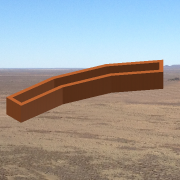
# Autodesk Inventor part: planter
Saved by Autodesk Inventor 2013 SP2 (Build 170200200, 200)
## iProperties
Created: 2014-01-03
Part Number: planter
Material: Wood (Cherry)
Document SubType Name: Modeling
Designer: Dave
Mass: 299055 g
Surface Area: 63083.1 cm^2
Volume: 598109 cm^3
Density: 0.5 g/cm^3
Author: Dave
Autodesk Inventor part; units mm, degrees
ref_plane "YZ Plane" through (0, 0, 0) normal (1, 0, 0) x (0, 1, 0)
ref_plane "XZ Plane" through (0, 0, 0) normal (0, 1, 0) x (-1, 0, 0)
ref_plane "XY Plane" through (0, 0, 0) normal (0, 0, 1) x (1, 0, 0)
sketch "Sketch3" plane through (0, 0, 0) normal (0, 1, 0) x (-1, 0, 0)
  line L0 (4876.8, 0) -> (4710.6271, -1262.2087)
  line L1 (4710.6271, -1262.2087) -> (4223.4327, -2438.4)
  line L2 (4223.4327, -2438.4) -> (3448.4184, -3448.4184)
  line L3 (3122.3395, -3122.3395) -> (3824.0693, -2207.8274)
  line L4 (3824.0693, -2207.8274) -> (4265.195, -1142.8556)
  line L5 (4265.195, -1142.8556) -> (4415.6548, 0)
  line L6 (4876.8, 0) -> (4415.6548, 0)
  line L7 (3448.4184, -3448.4184) -> (3122.3395, -3122.3395)
  line L8 (4776.121, 90.6289) -> (4876.8, 0)
  line L9 (3448.4184, -3448.4184) -> (3245.8, -3603.8929)
  point P0 (0, 0)
  point P1 (0, 0)
  dimension "d20" = 4876.8
  dimension "d25" = 457.2
  constraints: 20 end point, 2 point on line, 1 coincident, 1 horizontal, 8 other
  measures "d20" distance of L0.start point (0, 0)
  measures "d25" distance between parallel lines of L5 L0
extrude "Extrusion1" add sketch "Sketch3" along normal blind 457.2
sketch "Sketch4" plane through (0, 457.2, 0) normal (0, 1, 0) x (1, 0, 0)
  line L0 (-4710.6271, 1262.2087) -> (-4876.8, 0) projected
  line L1 (-4876.8, 0) -> (-4415.6548, 0) projected
  line L2 (-4415.6548, 0) -> (-4265.195, 1142.8556) projected
  line L3 (-4265.195, 1142.8556) -> (-3824.0693, 2207.8274) projected
  line L4 (-3824.0693, 2207.8274) -> (-3122.3395, 3122.3395) projected
  line L5 (-3122.3395, 3122.3395) -> (-3448.4184, 3448.4184) projected
  line L6 (-3448.4184, 3448.4184) -> (-4223.4327, 2438.4) projected
  line L7 (-4223.4327, 2438.4) -> (-4710.6271, 1262.2087) projected
  line L8 (-4145.7787, 2393.5664) -> (-3439.6, 3313.8764)
  line L9 (-3439.6, 3313.8764) -> (-3240.3296, 3114.606)
  line L10 (-3240.3296, 3114.606) -> (-3901.7233, 2252.661)
  line L11 (-3901.7233, 2252.661) -> (-4351.8068, 1166.0631)
  line L12 (-4351.8068, 1166.0631) -> (-4493.618, 88.9)
  line L13 (-4493.618, 88.9) -> (-4775.429, 88.9)
  line L14 (-4775.429, 88.9) -> (-4624.0153, 1239.0012)
  line L15 (-4624.0153, 1239.0012) -> (-4145.7787, 2393.5664)
  point P0 (0, 0)
  dimension "d24" = 88.9
  constraints: 16 end point, 7 other
  measures "d24" distance between parallel lines of L8 L6
extrude "Extrusion2" cut sketch "Sketch4" against normal blind 406.4 contours L8 L9 L10 L11 L12 L13 L14 L15
body "Solid1"
